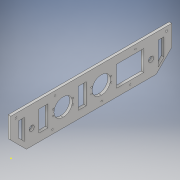
# Autodesk Inventor part: DriveTrainPlate
Saved by Autodesk Inventor 2017 (Build 210142000, 142)
## iProperties
Created: 2016-09-21
Part Number: DriveTrainPlate
Material: Generic
Document SubType Name: Modeling
Designer: RoboticsUser
Density: 1 g/cm^3
Appearance: Default
Mass: 175.92 g
Surface Area: 642.608 cm^2
Volume: 175.92 cm^3
Author: RoboticsUser
Autodesk Inventor part; units mm, degrees
ref_plane "YZ Plane" through (0, 0, 0) normal (1, 0, 0) x (0, 1, 0)
ref_plane "XZ Plane" through (0, 0, 0) normal (0, 1, 0) x (-1, 0, 0)
ref_plane "XY Plane" through (0, 0, 0) normal (0, 0, 1) x (1, 0, 0)
sketch "Sketch1" plane through (0, 0, 0) normal (1, 0, 0) x (0, 1, 0)
  line L0 (444.5, 0) -> (444.5, -2.1042)
  line L1 (0, -2.1042) -> (0, 0)
  line L2 (0, -74.1174) -> (0, -66.8433)
  line L3 (0, 0) -> (82.55, 0)
  line L4 (82.55, 0) -> (82.55, -393.7)
  line L5 (82.55, -393.7) -> (0, -393.7)
  line L6 (0, -393.7) -> (0, 0)
  point P0 (25.4, -50.8)
  point P1 (25.4, -342.9)
  dimension "d2" = 82.55
  dimension "d3" = 393.7
  dimension "d4" = 50.8
  dimension "d5" = 25.4
  dimension "d6" = 50.8
  dimension "d7" = 25.4
  constraints: 14 end point, 3 parallel, 1 horizontal, 1 perpendicular, 1 point on line
  measures "d2" distance of L4.end L5.end
  measures "d3" distance of L3.end L4.end
  measures "d4" distance from line of L3 point (25.4, -50.8)
  measures "d5" distance from line of L6 point (25.4, -50.8)
  measures "d6" distance from line of L5 point (25.4, -342.9)
  measures "d7" distance from line of L6 point (25.4, -342.9)
extrude "Extrusion1" add sketch "Sketch1" along normal blind 6.35
sketch "Sketch3" plane through (6.35, 0, 0) normal (1, 0, 0) x (0, 0, -1)
  point P0 (0, 0)
sketch "Sketch4" plane through (6.35, 0, 0) normal (1, 0, 0) x (0, 0, -1)
  point P0 (0, 0)
chamfer "Chamfer1" distance 38.1 angle 45 1 edges at (3.175, 0, 0)
chamfer "Chamfer2" distance 38.1 angle 45 1 edges at (3.175, 0, -393.7)
sketch "Sketch5" plane through (0, 0, 0) normal (-1, 0, 0) x (0, 0, 1)
  line L0 (0, 82.55) -> (-393.7, 82.55) projected
  line L1 (-355.6, 0) -> (-393.7, 38.1) projected
  line L2 (-355.6, 0) -> (-38.1, 0) projected
  line L3 (0, 38.1) -> (-38.1, 0) projected
  line L4 (0, 38.1) -> (0, 82.55) projected
  line L5 (0, 82.55) -> (-393.7, 82.55) projected
  line L6 (-393.7, 82.55) -> (-393.7, 38.1) projected
  point P0 (0, 0)
  point P1 (-342.9, 38.1)
  point P2 (-50.8, 38.1)
  dimension "d16" = 50.8
  dimension "d17" = 38.1
  dimension "d18" = 38.1
  dimension "d19" = 50.8
  measures "d16" distance from line of L6 point (-342.9, 38.1)
  measures "d17" distance from line of point (-342.9, 38.1) L2
  measures "d18" distance from line of L2 point (-50.8, 38.1)
  measures "d19" distance from line of L4 point (-50.8, 38.1)
hole "Hole1" at (0, 38.1, -342.9) at (0, 38.1, -50.8) direction (1, 0, 0) diameter 12.7254 end through all
sketch "Sketch7" plane through (0, 0, 0) normal (-1, 0, 0) x (0, 0, 1)
  line L0 (-38.1, 0) -> (-355.6, 0) projected
  line L1 (-393.7, 82.55) -> (-393.7, 38.1) projected
  line L2 (0, 38.1) -> (0, 82.55) projected
  line L3 (0, 82.55) -> (-393.7, 82.55) projected
  point P0 (0, 0)
  point P1 (-298.45, 10.0076)
  point P2 (-95.25, 10.0076)
  point P3 (-12.7, 78.8924)
  point P4 (-381, 78.8924)
  dimension "d42" = 10.0076
  dimension "d43" = 95.25
  dimension "d44" = 95.25
  dimension "d45" = 3.6576
  dimension "d46" = 12.7
  dimension "d47" = 12.7
  dimension "d82" = 3.6576
  measures "d42" distance from line of L0 point (-298.45, 10.008)
  measures "d43" distance from line of L1 point (-298.45, 10.008)
  measures "d44" distance from line of L2 point (-95.25, 10.008)
  measures "d45" distance from line of L3 point (-12.7, 78.892)
  measures "d46" distance from line of point (-12.7, 78.892) L2
  measures "d47" distance from line of L1 point (-381, 78.892)
  measures "d82" distance from line of L3 point (-381, 78.892)
hole "Hole3" at (0, 78.8924, -381) at (0, 78.8924, -12.7) direction (1, 0, 0) diameter 4.7752 end through all
sketch "Sketch8" plane through (0, 0, 0) normal (-1, 0, 0) x (0, 0, 1)
  line L0 (0, 38.1) -> (0, 82.55) projected
  line L1 (0, 82.55) -> (-393.7, 82.55) projected
  line L2 (-355.6, 0) -> (-38.1, 0) projected
  line L3 (-393.7, 38.1) -> (-393.7, 82.55) projected
  point P0 (0, 0)
  point P1 (-171.45, 78.8924)
  point P2 (-222.25, 10.0076)
  dimension "d57" = 10.0076
  dimension "d128" = 222.25
  measures "d57" distance from line of L2 point (-222.25, 10.008)
  measures "d128" distance from line of L0 point (-222.25, 10.008)
hole "Hole4" at (0, 10.0076, -222.25) direction (1, 0, 0) diameter 3.556 end through all
sketch "Sketch10" plane through (0, 0, 0) normal (-1, 0, 0) x (0, 0, 1)
  circle A0 centre (-222.25, 44.45) radius 1.778
  circle A1 centre (-127, 44.45) radius 1.778
  line L0 (-393.7, 82.55) -> (0, 82.55) projected
  line L1 (-114.3619, 67.6125) -> (-112.4836, 67.6125)
  point P0 (0, 0)
  point P1 (-220.472, 44.45)
  point P2 (-128.778, 44.45)
  dimension "d108" = 38.1
  dimension "d109" = 38.1
  constraints: 2 end point, 2 horizontal alignment, 1 horizontal, 4 other
  measures "d108" distance from line of L0 point (-127, 44.45)
  measures "d109" distance from line of L0 point (-222.25, 44.45)
hole "Hole6" at (0, 44.45, -127) at (0, 44.45, -220.472) at (0, 44.45, -128.778) at (0, 44.45, -222.25) direction (1, 0, 0) diameter 43.18 end through all
sketch "Sketch14" plane through (6.35, 0, 0) normal (1, 0, 0) x (0, 0, -1)
  arc A0 (127.889, 66.0217) -> (127.889, 22.8783) centre (127, 44.45) ccw projected
  arc A1 (127.889, 22.8783) -> (127.889, 66.0217) centre (128.778, 44.45) ccw projected
  arc A2 (221.361, 66.0217) -> (221.361, 22.8783) centre (220.472, 44.45) ccw projected
  arc A3 (221.361, 22.8783) -> (221.361, 66.0217) centre (222.25, 44.45) ccw projected
  line L0 (127.889, 66.0217) -> (127.889, 22.8783)
  line L1 (96.03, 44.45) -> (156.5626, 44.45)
  line L2 (221.361, 66.0217) -> (221.361, 22.8783)
  line L3 (190.5646, 36.322) -> (248.6345, 36.322)
  line L4 (127.889, 44.45) -> (103.886, 44.45)
  line L5 (103.886, 44.45) -> (103.886, 51.4604)
  line L6 (103.886, 51.4604) -> (103.886, 44.45)
  line L7 (103.886, 44.45) -> (103.886, 37.4396)
  line L8 (127.889, 44.45) -> (151.892, 44.45)
  line L9 (151.892, 44.45) -> (151.892, 37.4396)
  line L10 (151.892, 44.45) -> (151.892, 51.4604)
  line L11 (221.361, 51.4604) -> (197.358, 51.4604)
  line L12 (221.361, 51.4604) -> (245.364, 51.4604)
  line L13 (221.361, 37.4396) -> (197.358, 37.4396)
  line L14 (221.361, 37.4396) -> (245.364, 37.4396)
  circle A4 centre (103.886, 37.4396) radius 1.7526
  circle A5 centre (103.886, 51.4604) radius 1.7526
  circle A6 centre (151.892, 51.4604) radius 1.7526
  circle A7 centre (151.892, 37.4396) radius 1.7526
  circle A8 centre (197.358, 51.4604) radius 1.7526
  circle A9 centre (197.358, 37.4396) radius 1.7526
  circle A10 centre (245.364, 37.4396) radius 1.7526
  circle A11 centre (245.364, 51.4604) radius 1.7526
  point P0 (0, 0)
  dimension "d113" = 24.003
  dimension "d114" = 7.0104
  dimension "d115" = 7.0104
  dimension "d116" = 24.003
  dimension "d117" = 24.003
  dimension "d118" = 24.003
  dimension "d119" = 3.5052
  dimension "d120" = 3.5052
  dimension "d121" = 3.5052
  dimension "d122" = 3.5052
  dimension "d123" = 3.5052
  constraints: 30 end point, 8 centre point, 8 coincident, 6 point on line, 5 horizontal, 3 perpendicular, 3 vertical, 1 collinear, 1 midpoint
  measures "d113" distance of L4.start L4.end
  measures "d114" distance of L4.end L5.end
  measures "d115" distance of L4.end L7.end
  measures "d116" distance of L4.start L8.end
  measures "d117" distance of L11.start L11.end
  measures "d118" distance of L11.start L12.end
  measures "d119" diameter of A4
  measures "d120" diameter of A5
  measures "d121" diameter of A6
  measures "d122" diameter of A7
  measures "d123" diameter of A8
extrude "Extrusion2" cut sketch "Sketch14" against normal blind 25.4 contours A9 L3 | A10 L3 | A9 L3 | L3 A10 | A4 | A5 | A6 | A7 | A8 | A11
thicken "Thicken1" operation add thickness 6.35 both sides no extend neighbours yes toward (0, 1, 0) faces at (2.1167, 82.55, -131.2333)
sketch "Sketch16" plane through (6.35, 0, 0) normal (1, 0, 0) x (0, 0, -1)
  line L0 (393.7, 88.9) -> (0, 88.9) projected
  line L1 (42.6019, 88.9) -> (52.7619, 88.9)
  line L2 (52.7619, 88.9) -> (52.7619, 78.74)
  line L3 (31.75, 78.74) -> (107.95, 78.74)
  line L4 (31.75, 78.74) -> (107.95, 78.74) construction
  point P0 (0, 0)
  dimension "d131" = 10.16
  dimension "d132" = 10.16
  dimension "d133" = 76.2
  constraints: 8 end point, 2 horizontal, 2 point on line, 1 collinear, 1 perpendicular
  measures "d131" distance of L1.start L1.end
  measures "d132" distance of L1.end L2.end
  measures "d133" distance of L3.start L3.end
sketch "Sketch17" plane through (6.35, 0, 0) normal (1, 0, 0) x (0, 0, -1)
  circle A0 centre (139.7, 78.74) radius 1.778
  line L0 (393.7, 38.1) -> (393.7, 88.9) projected
  line L1 (393.7, 78.74) -> (304.8, 78.74)
  line L2 (393.7, 78.74) -> (482.6, 78.74) construction
  circle A1 centre (304.8, 78.74) radius 1.778
  point P0 (0, 0)
  dimension "d135" = 3.556
  dimension "d136" = 88.9
  dimension "d138" = 3.556
  constraints: 4 end point, 3 coincident, 2 centre point, 1 collinear, 1 horizontal, 1 perpendicular, 1 point on line
  measures "d135" diameter of A0
  measures "d136" distance of L1.start L1.end
  measures "d138" diameter of A1
sketch "Sketch18" plane through (6.35, 0, 0) normal (1, 0, 0) x (0, 0, -1)
  line L0 (0, 0) -> (0, 10.0076)
  line L1 (0, 0) -> (10.0076, 0) construction
  line L2 (0, 10.0076) -> (101.6, 10.0076)
  line L3 (0, 10.0076) -> (101.6, 10.0076) construction
  line L4 (393.7, 10.0076) -> (292.1, 10.0076)
  line L5 (393.7, 10.0076) -> (495.3, 10.0076) construction
  circle A0 centre (101.6, 10.0076) radius 2.3876
  circle A1 centre (292.1, 10.0076) radius 2.3876
  dimension "d139" = 10.0076
  dimension "d141" = 101.6
  dimension "d143" = 101.6
  dimension "d145" = 4.7752
  dimension "d146" = 4.7752
  constraints: 12 end point, 5 horizontal, 4 coincident, 3 equal length, 2 centre point, 1 vertical
  measures "d139" distance of L0.start L0.end
  measures "d141" distance of L0.end L2.end
  measures "d143" distance of L4.start L4.end
  measures "d145" diameter of A0
  measures "d146" diameter of A1
hole "Hole10" at (6.35, 78.74, -107.95) direction (-1, 0, 0) diameter 3.556 depth 25.4 tip angle 118
hole "Hole11" at (6.35, 78.74, -304.8) direction (-1, 0, 0) diameter 3.556 depth 25.4 tip angle 118
hole "Hole12" at (6.35, 10.0076, -292.1) direction (-1, 0, 0) diameter 3.556 depth 25.4 tip angle 118
hole "Hole13" at (6.35, 10.0076, -101.6) direction (-1, 0, 0) diameter 3.556 depth 25.4 tip angle 118
sketch "Sketch19" plane through (6.35, 0, 0) normal (1, 0, 0) x (0, 0, -1)
  point P0 (0, 0)
sketch "Sketch20" plane through (6.35, 0, 0) normal (1, 0, 0) x (0, 0, -1)
  line L0 (0, 88.9) -> (0, 38.1) projected
  line L1 (38.1, 0) -> (0, 38.1) projected
  line L2 (38.1, 0) -> (355.6, 0) projected
  line L3 (393.7, 38.1) -> (355.6, 0) projected
  line L4 (393.7, 38.1) -> (393.7, 88.9) projected
  line L5 (393.7, 88.9) -> (0, 88.9) projected
  line L6 (0, 63.5) -> (19.05, 63.5)
  line L7 (19.05, 88.9) -> (19.05, 69.85)
  line L8 (56.4869, 0) -> (56.4869, 19.05)
  circle A0 centre (50.8, 38.1) radius 6.3627 projected
  circle A1 centre (50.8, 38.1) radius 6.3627 projected
  line L9 (44.4412, 37.8775) -> (33.0112, 37.8775)
  line L10 (50.5074, 44.456) -> (50.5074, 55.886)
  line L11 (57.1622, 38.1805) -> (68.5922, 38.1805)
  circle A2 centre (103.886, 37.4396) radius 1.7526 projected
  line L12 (102.1334, 37.4396) -> (90.7034, 37.4396)
  line L13 (80.4606, 88.9) -> (80.4606, 69.85)
  line L14 (68.5922, 69.85) -> (90.7034, 69.85)
  line L15 (90.7034, 69.85) -> (90.7034, 19.05)
  line L16 (90.7034, 19.05) -> (68.5922, 19.05)
  line L17 (68.5922, 19.05) -> (68.5922, 69.85)
  line L18 (19.05, 69.85) -> (33.0112, 69.85)
  line L19 (33.0112, 69.85) -> (33.0112, 33.0112)
  line L20 (33.0112, 33.0112) -> (19.05, 33.0112)
  line L21 (19.05, 33.0112) -> (19.05, 69.85)
  line L22 (19.05, 33.0112) -> (33.0112, 33.0112)
  line L23 (33.0112, 33.0112) -> (33.0112, 19.05)
  line L24 (33.0112, 19.05) -> (19.05, 33.0112)
  line L25 (33.0112, 19.05) -> (33.0112, 33.0112)
  line L26 (19.05, 33.0112) -> (33.0112, 33.0112)
  line L27 (19.05, 33.0112) -> (33.0112, 19.05)
  line L28 (33.0112, 33.0112) -> (33.0112, 69.85)
  line L29 (33.0112, 69.85) -> (19.05, 69.85)
  line L30 (19.05, 69.85) -> (19.05, 33.0112)
  point P0 (0, 0)
  dimension "d183" = 19.05
  dimension "d184" = 19.05
  dimension "d185" = 19.05
  dimension "d186" = 11.43
  dimension "d187" = 11.43
  dimension "d188" = 11.43
  dimension "d189" = 11.43
  dimension "d190" = 19.05
  constraints: 50 end point, 7 horizontal, 6 perpendicular, 6 point on circle, 5 equal length, 4 vertical, 3 point on line, 1 horizontal alignment, 1 midpoint, 1 other
  measures "d183" distance of L6.start L6.end
  measures "d184" distance of L7.start L7.end
  measures "d185" distance of L8.start L8.end
  measures "d186" distance of L9.start L9.end
  measures "d187" distance of L10.start L10.end
  measures "d188" distance of L11.start L11.end
  measures "d189" distance of L12.start L12.end
  measures "d190" distance of L13.start L13.end
extrude "Extrusion3" cut sketch "Sketch20" against normal blind 25.4 contours L14 L15 L16 L17
extrude "Extrusion4" cut sketch "Sketch20" against normal blind 25.4 contours L21 L18 L19 L20 | L20 L23 L24
sketch "Sketch21" plane through (6.35, 0, 0) normal (1, 0, 0) x (0, 0, -1)
  circle A0 centre (151.892, 51.4604) radius 1.7526 projected
  line L0 (38.1, 0) -> (355.6, 0) projected
  circle A1 centre (197.358, 51.4604) radius 1.7526 projected
  line L1 (393.7, 88.9) -> (0, 88.9) projected
  line L2 (0, 88.9) -> (393.7, 88.9) projected
  line L3 (175.7731, 88.9) -> (175.7731, 69.85)
  line L4 (153.6446, 51.4604) -> (165.0746, 51.4604)
  circle A2 centre (197.358, 51.4604) radius 1.7526 projected
  line L5 (195.6055, 51.4771) -> (184.1755, 51.4771)
  line L6 (355.6, 0) -> (38.1, 0) projected
  line L7 (175.7731, 0) -> (175.7731, 19.05)
  line L8 (165.0746, 69.85) -> (184.1755, 69.85)
  line L9 (184.1755, 69.85) -> (184.1755, 19.05)
  line L10 (184.1755, 19.05) -> (165.0746, 19.05)
  line L11 (165.0746, 19.05) -> (165.0746, 69.85)
  circle A3 centre (245.364, 51.4604) radius 1.7526 projected
  circle A4 centre (245.364, 37.4396) radius 1.7526 projected
  circle A5 centre (342.9, 38.1) radius 6.3627 projected
  line L12 (267.1323, 0) -> (267.1323, 19.05)
  line L13 (267.1323, 88.9) -> (267.1323, 69.85)
  line L14 (247.1166, 51.4604) -> (258.5466, 51.4604)
  line L15 (336.5373, 38.1) -> (325.1073, 38.1)
  line L16 (258.5466, 69.85) -> (325.1073, 69.85)
  line L17 (325.1073, 69.85) -> (325.1073, 19.05)
  line L18 (325.1073, 19.05) -> (258.5466, 19.05)
  line L19 (258.5466, 19.05) -> (258.5466, 69.85)
  point P0 (0, 0)
  dimension "d195" = 19.05
  dimension "d196" = 11.43
  dimension "d197" = 11.43
  dimension "d198" = 19.05
  dimension "d199" = 19.05
  dimension "d200" = 19.05
  dimension "d201" = 11.43
  dimension "d202" = 11.43
  constraints: 32 end point, 6 horizontal, 6 perpendicular, 4 parallel, 4 point on line, 3 horizontal alignment, 7 other
  measures "d195" distance of L3.start L3.end
  measures "d196" distance of L4.start L4.end
  measures "d197" distance of L5.start L5.end
  measures "d198" distance of L7.start L7.end
  measures "d199" distance of L12.start L12.end
  measures "d200" distance of L13.start L13.end
  measures "d201" distance of L14.start L14.end
  measures "d202" distance of L15.start L15.end
extrude "Extrusion5" cut sketch "Sketch21" against normal blind 25.4 contours L10 L11 L8 L9
extrude "Extrusion6" cut sketch "Sketch21" against normal blind 25.4 contours L18 L19 L16 L17
sketch "Sketch22" plane through (6.35, 0, 0) normal (1, 0, 0) x (0, 0, -1)
  line L0 (393.7, 38.1) -> (393.7, 88.9) projected
  line L1 (361.8045, 88.9) -> (361.8045, 69.85)
  circle A0 centre (342.9, 38.1) radius 6.3627 projected
  line L2 (349.2627, 38.1) -> (360.6927, 38.1)
  line L3 (393.7, 39.2414) -> (374.65, 39.2414)
  line L4 (360.6927, 69.85) -> (374.65, 69.85)
  line L5 (374.65, 69.85) -> (374.65, 27.244)
  line L6 (374.65, 27.244) -> (360.6927, 27.244)
  line L7 (360.6927, 27.244) -> (360.6927, 69.85)
  line L8 (360.6927, 27.244) -> (360.6927, 13.2867)
  line L9 (360.6927, 13.2867) -> (374.65, 27.244)
  line L10 (355.6, 0) -> (393.7, 38.1) projected
  point P0 (0, 0)
  dimension "d207" = 19.05
  dimension "d208" = 11.43
  dimension "d209" = 19.05
  constraints: 18 end point, 3 parallel, 2 horizontal, 2 perpendicular, 2 vertical, 1 horizontal alignment, 1 point on line, 1 other
  measures "d207" distance of L1.start L1.end
  measures "d208" distance of L2.start L2.end
  measures "d209" distance of L3.start L3.end
extrude "Extrusion7" cut sketch "Sketch22" against normal blind 25.4 contours L4 L5 L6 L7 | L6 L9 L8
chamfer "Chamfer5" distance 3.175 angle 45 3 edges at (0, 78.74, -303.022) (0, 10.0076, -224.028) (0, 78.74, -106.172)
body "Solid1"
